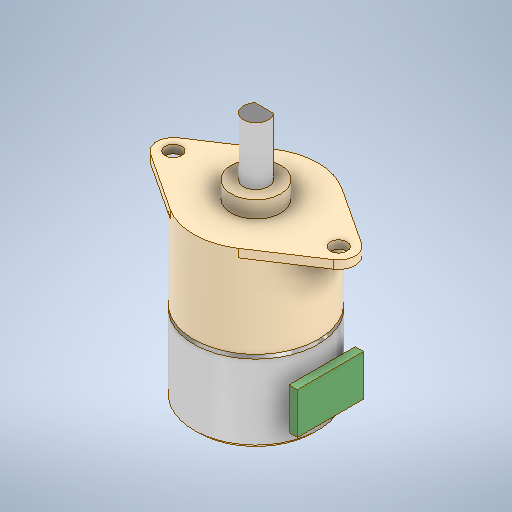
# Autodesk Inventor part: Stepper-D15-S18
Saved by Autodesk Inventor 2025.3 (Build 293356000, 356)
## iProperties
Created: 2025-06-27
Part Number: Stepper-D15-S18
Material: 一般
Document SubType Name: Modeling
Designer: yamashita1
Density: 1 g/cm^3
Appearance: 滑らか - オフホワイト
Author: yamashita1
Autodesk Inventor part; units mm, degrees
ref_plane "XZ Plane" through (0, 0, 0) normal (0, 1, 0) x (-1, 0, 0)
ref_plane "XY Plane" through (0, 0, 0) normal (0, 0, 1) x (1, 0, 0)
sketch "スケッチ2" plane through (0, 0, 0) normal (0, 1, 0) x (-1, 0, 0)
  line L0 (0, 0) -> (7, 0)
  line L1 (7, 0) -> (7.5, 0.5)
  line L2 (7.5, 0.5) -> (7.5, 9.5)
  line L3 (7.5, 9.5) -> (7, 10)
  line L4 (7, 10) -> (0, 10)
  line L5 (0, 10) -> (0, 0)
  dimension "d0" = 7.5
  dimension "d1" = 10
  dimension "d2" = 135
  dimension "d3" = 0.5
  constraints: 12 end point, 3 perpendicular, 1 horizontal, 1 parallel, 1 vertical alignment
  measures "d0" distance between parallel lines of L2 L5
  measures "d1" distance of L4.end L0.start
  measures "d2" angle of L0 L1
  measures "d3" horizontal distance of L1.end L0.end
revolve "回転1" add sketch "スケッチ2" angle 360 about axis through (0, 0, 10) along (0, 0, -1)
sketch "スケッチ3" plane through (0, 0, 10) normal (0, 0, 1) x (1, 0, 0)
  point P0 (0, 0)
sketch "スケッチ4" plane through (0, 0, 10) normal (0, 0, 1) x (1, 0, 0)
  circle A0 centre (0, 0) radius 7.5
  circle A1 centre (0, 0) radius 7.5 projected
  constraints: 2 concentric, 1 centre point
extrude "押し出し1" add sketch "スケッチ4" along normal blind 11
sketch "スケッチ5" plane through (0, 0, 21) normal (0, 0, 1) x (1, 0, 0)
  line L0 (-15.0014, 0) -> (15.0014, 0) construction
  line L1 (0, 10.7122) -> (0, -10.7122) construction
  circle A0 centre (-10, 0) radius 1
  circle A1 centre (10, 0) radius 1
  circle A2 centre (-10, 0) radius 2
  circle A3 centre (10, 0) radius 2
  circle A4 centre (0, 0) radius 7.5
  circle A5 centre (0, 0) radius 7.5 projected
  line L2 (-11.1, 1.6703) -> (-4.125, 6.2637)
  line L3 (-11.1, -1.6703) -> (-4.125, -6.2637)
  line L4 (4.125, -6.2637) -> (11.1, -1.6703)
  line L5 (11.1, 1.6703) -> (4.125, 6.2637)
  point P0 (0, 0)
  point P1 (-4.125, -6.2637)
  dimension "d7" = 2
  dimension "d8" = 20
  dimension "d9" = 4
  constraints: 12 end point, 7 point on circle, 6 tangent, 4 centre point, 4 coincident, 2 equal radius, 2 midpoint, 2 point on line, 1 horizontal, 1 perpendicular, 1 symmetric about line, 7 other
  measures "d7" diameter of A0
  measures "d8" distance of A1.centre A0.centre
  measures "d9" diameter of A2
extrude "押し出し2" add sketch "スケッチ5" against normal blind 1 contours A2 | A2 L2 A4 L3 | L5 A3 L4 A4 | A3
sketch "スケッチ6" plane through (0, 0, 21) normal (0, 0, 1) x (1, 0, 0)
  circle A0 centre (0, 0) radius 3
  dimension "d12" = 6
  constraints: 1 centre point, 1 coincident
  measures "d12" diameter of A0
extrude "押し出し3" add sketch "スケッチ6" along normal blind 2
sketch "スケッチ7" plane through (0, 0, 23) normal (0, 0, 1) x (1, 0, 0)
  circle A0 centre (0, 0) radius 1.5
  dimension "d15" = 3
  constraints: 1 centre point, 1 coincident
  measures "d15" diameter of A0
extrude "押し出し4" add sketch "スケッチ7" along normal blind 7
sketch "スケッチ8" plane through (0, 0, 30) normal (0, 0, 1) x (1, 0, 0)
  circle A0 centre (0, 0) radius 1.5
  circle A1 centre (0, 0) radius 1.5 projected
  line L0 (-1.118, 1) -> (1.118, 1)
  dimension "d19" = 2.5
  constraints: 2 end point, 2 point on circle, 1 centre point, 1 coincident, 1 concentric, 1 horizontal
extrude "押し出し5" cut sketch "スケッチ8" against normal blind 6.5 contours L0 A0 picked at (-0.0599, 1.1631)
ref_plane "作業平面1" through (8, 0, 0) normal (1, 0, 0) x (0, 1, 0)
sketch "スケッチ9" plane through (8, 0, 0) normal (1, 0, 0) x (0, 1, 0)
  line L0 (-4, 7.5) -> (4, 7.5)
  line L1 (4, 7.5) -> (4, 2.5)
  line L2 (4, 2.5) -> (-4, 2.5)
  line L3 (-4, 2.5) -> (-4, 7.5)
  point P0 (0, 0)
  point P1 (0, 2.5)
  dimension "d23" = 8
  dimension "d24" = 5
  dimension "d25" = 2.5
  constraints: 8 end point, 2 parallel, 1 horizontal, 1 midpoint, 1 perpendicular, 1 vertical alignment
  measures "d23" distance of L1.end L2.end
  measures "d24" distance of L0.end L1.end
  measures "d25" distance from line of point (0, 0) L2
extrude "押し出し6" add sketch "スケッチ9" along normal blind 1
